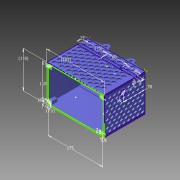
# Autodesk Inventor part: Box
Saved by Autodesk Inventor 2015 (Build 190159000, 159)
## iProperties
Created: 2015-04-29
Part Number: Box
Material: ABS Plastic
Document SubType Name: Modeling
Designer: Akovo_000
Mass: 201.139 g
Surface Area: 2118.44 cm^2
Volume: 189.753 cm^3
Density: 1.06 g/cm^3
Appearance: Smooth - White
Author: Akovo_000
Autodesk Inventor part; units mm, degrees
(part 1 of 2)
ref_plane "YZ Plane" through (0, 0, 0) normal (1, 0, 0) x (0, 1, 0)
ref_plane "XZ Plane" through (0, 0, 0) normal (0, 1, 0) x (-1, 0, 0)
ref_plane "XY Plane" through (0, 0, 0) normal (0, 0, 1) x (1, 0, 0)
sketch "BasicBox" plane through (0, 0, 0) normal (0, 1, 0) x (-1, 0, 0)
  line L0 (88.1704, 47.7191) -> (-86.8296, 47.7191)
  line L1 (-86.8296, 47.7191) -> (-86.8296, -62.2809)
  line L2 (-86.8296, -62.2809) -> (88.1704, -62.2809)
  line L3 (88.1704, -62.2809) -> (88.1704, 47.7191)
  line L4 (92.1704, 51.7191) -> (-90.8296, 51.7191)
  line L5 (-90.8296, 51.7191) -> (-90.8296, -66.2809)
  line L6 (-90.8296, -66.2809) -> (92.1704, -66.2809)
  line L7 (92.1704, -66.2809) -> (92.1704, 51.7191)
  line L8 (88.1704, 47.7191) -> (88.1704, 48.5191) construction
  line L9 (88.1704, 47.7191) -> (88.9704, 47.7191) construction
  line L10 (88.1704, -62.2809) -> (88.1704, -63.0809) construction
  line L11 (88.1704, -62.2809) -> (88.9704, -62.2809) construction
  line L12 (-86.8296, -62.2809) -> (-86.8296, -63.0809) construction
  line L13 (-86.8296, 47.7191) -> (-86.8296, 48.5191) construction
  line L14 (-86.8296, 47.7191) -> (-87.6296, 47.7191) construction
  line L15 (-86.8296, -62.2809) -> (-87.6296, -62.2809) construction
  line L16 (-87.6296, -63.0809) -> (-87.6296, -62.2809)
  line L17 (-87.6296, 48.5191) -> (-86.8296, 48.5191)
  line L18 (88.9704, 48.5191) -> (88.9704, -62.2809)
  line L19 (88.9704, -63.0809) -> (88.1704, -63.0809)
  line L20 (88.9704, 47.7191) -> (92.1704, 47.7191) construction
  line L21 (88.1704, 48.5191) -> (88.1704, 51.7191) construction
  line L22 (-86.8296, 48.5191) -> (88.9704, 48.5191)
  line L23 (-87.6296, 47.7191) -> (-87.6296, 48.5191)
  line L24 (-87.6296, -62.2809) -> (-87.6296, 47.7191)
  line L25 (-86.8296, -63.0809) -> (-87.6296, -63.0809)
  line L26 (88.9704, -62.2809) -> (88.9704, -63.0809)
  line L27 (88.1704, -63.0809) -> (-86.8296, -63.0809)
  line L28 (88.9704, -62.2809) -> (92.1704, -62.2809) construction
  line L29 (88.1704, -63.0809) -> (88.1704, -66.2809) construction
  line L30 (-87.6296, 47.7191) -> (-90.8296, 47.7191) construction
  line L31 (-86.8296, 48.5191) -> (-86.8296, 51.7191) construction
  line L32 (-87.6296, -62.2809) -> (-90.8296, -62.2809) construction
  line L33 (-86.8296, -63.0809) -> (-86.8296, -66.2809) construction
  line L34 (-76.8296, -62.2809) -> (-76.8296, -52.2809)
  line L35 (-76.8296, -52.2809) -> (-86.8296, -52.2809)
  line L36 (-76.8296, 47.7191) -> (-76.8296, 37.7191)
  line L37 (-76.8296, 37.7191) -> (-86.8296, 37.7191)
  line L38 (78.9704, 47.7191) -> (78.9704, 37.7191)
  line L39 (78.9704, 37.7191) -> (88.1704, 37.7191)
  line L40 (88.9704, -52.2809) -> (78.9704, -52.2809)
  line L41 (78.9704, -52.2809) -> (78.9704, -62.2809)
  line L42 (78.9704, 47.7191) -> (78.9704, 51.7191)
  line L43 (88.1704, 37.7191) -> (92.1704, 37.7191)
  line L44 (78.9704, -62.2809) -> (78.9704, -66.2809)
  line L45 (88.9704, -52.2809) -> (92.1704, -52.2809)
  line L46 (-80.7674, -55.2809) -> (-78.7467, -58.7809)
  line L47 (-78.7467, -58.7809) -> (-80.7674, -62.2809)
  line L48 (-80.7674, -62.2809) -> (-84.8089, -62.2809)
  line L49 (-84.8089, -62.2809) -> (-86.8296, -58.7809)
  line L50 (-86.8296, -58.7809) -> (-84.8089, -55.2809)
  line L51 (-84.8089, -55.2809) -> (-80.7674, -55.2809)
  line L52 (-80.7674, 47.7191) -> (-78.7467, 44.2191)
  line L53 (-78.7467, 44.2191) -> (-80.7674, 40.7191)
  line L54 (-80.7674, 40.7191) -> (-84.8089, 40.7191)
  line L55 (-84.8089, 40.7191) -> (-86.8296, 44.2191)
  line L56 (-86.8296, 44.2191) -> (-84.8089, 47.7191)
  line L57 (-84.8089, 47.7191) -> (-80.7674, 47.7191)
  line L58 (86.1497, 47.7191) -> (88.1704, 44.2191)
  line L59 (88.1704, 44.2191) -> (86.1497, 40.7191)
  line L60 (86.1497, 40.7191) -> (82.1082, 40.7191)
  line L61 (82.1082, 40.7191) -> (80.0875, 44.2191)
  line L62 (80.0875, 44.2191) -> (82.1082, 47.7191)
  line L63 (82.1082, 47.7191) -> (86.1497, 47.7191)
  line L64 (86.1497, -55.2809) -> (88.1704, -58.7809)
  line L65 (88.1704, -58.7809) -> (86.1497, -62.2809)
  line L66 (86.1497, -62.2809) -> (82.1082, -62.2809)
  line L67 (82.1082, -62.2809) -> (80.0875, -58.7809)
  line L68 (80.0875, -58.7809) -> (82.1082, -55.2809)
  line L69 (82.1082, -55.2809) -> (86.1497, -55.2809)
  circle A0 centre (84.129, 44.2191) radius 2
  circle A1 centre (84.129, -58.7809) radius 2
  circle A2 centre (-82.7881, -58.7809) radius 2
  circle A3 centre (-82.7881, 44.2191) radius 2
  point P0 (0, 0)
  dimension "d2" = 110
  dimension "d3" = 175
  dimension "d4" = 4
  dimension "d68" = 0.8
  dimension "d71" = 4
  dimension "d94" = 10
  dimension "d95" = 183
  dimension "d96" = 118
  dimension "d97" = 7
  dimension "d98" = 0
  dimension "d101" = 0
  dimension "d102" = 4
  dimension "d105" = 0
  dimension "d106" = 0
  dimension "d109" = 7.5
  dimension "d110" = 8.0414
  constraints: 140 end point, 29 point on line, 22 perpendicular, 14 equal length, 9 parallel, 6 vertical, 5 collinear, 4 centre point, 4 coincident, 4 horizontal, 3 equal radius, 52 other
  measures "d2" distance of L28.end L20.end
  measures "d3" distance of L29.end L33.end
  measures "d4" distance of L6.end L28.end
  measures "d68" distance of L16.start L12.end
  measures "d71" distance of L6.end L29.end
  measures "d94" distance of L34.start L34.end
  measures "d95" distance between parallel lines of L7 L5
  measures "d96" distance between parallel lines of L4 L6
  measures "d97" distance between parallel lines of L51 L48
  measures "d98" distance from line of L1 L49.end
  measures "d101" distance from line of L3 L64.end
  measures "d102" diameter of A0
  measures "d105" distance from line of L1 L55.end
  measures "d106" distance from line of L3 L58.end
  measures "d109" distance from line of L6 point (84.129, -58.781)
  measures "d110" distance from line of L7 point (84.129, -58.781)
extrude "Extrusion1" add sketch "BasicBox" along normal blind 131 contours L0 L42 L22 L18 L43 L3 | L43 L18 L40 L3 | L0 L1 L2 L44 L27 L25 L16 L24 L23 L17 L22 L42 | L40 L18 L26 L19 L27 L44 L2 L3 | L43 L7 L45 L18 | L18 L22 L42 L4 L7 L43 | L22 L17 L23 L24 L16 L25 L27 L44 L6 L5 L4 L42 | L45 L7 L6 L44 L27 L19 L26 L18
sketch "LongerHonycomb" plane through (-92.1704, 0, 51.7191) normal (0, 0, 1) x (1, 0, 0)
  line L0 (0, 131) -> (183, 131)
  line L1 (183, 131) -> (183, 0)
  line L2 (183, 0) -> (0, 0)
  line L3 (0, 0) -> (0, 131)
  line L4 (0, 131) -> (183, 131) projected
  line L5 (179, 131) -> (179, 0)
  line L6 (4, 131) -> (4, 0)
  line L7 (179, 131) -> (4, 131) projected
  line L8 (4, 0) -> (179, 0) projected
  line L9 (17.3923, 116) -> (10.4641, 116)
  line L10 (10.4641, 116) -> (7, 122)
  line L11 (7, 122) -> (10.4641, 128)
  line L12 (10.4641, 128) -> (17.3923, 128)
  line L13 (17.3923, 128) -> (20.8564, 122)
  line L14 (20.8564, 122) -> (17.3923, 116)
  line L15 (32.4034, 114) -> (28.9393, 108)
  line L16 (28.9393, 108) -> (22.0111, 108)
  line L17 (22.0111, 108) -> (18.547, 114)
  line L18 (18.547, 114) -> (22.0111, 120)
  line L19 (22.0111, 120) -> (28.9393, 120)
  line L20 (28.9393, 120) -> (32.4034, 114)
  line L21 (40.4923, 116) -> (33.5641, 116)
  line L22 (33.5641, 116) -> (30.1, 122)
  line L23 (30.1, 122) -> (33.5641, 128)
  line L24 (33.5641, 128) -> (40.4923, 128)
  line L25 (40.4923, 128) -> (43.9564, 122)
  line L26 (43.9564, 122) -> (40.4923, 116)
  line L27 (55.5034, 114) -> (52.0393, 108)
  line L28 (52.0393, 108) -> (45.1111, 108)
  line L29 (45.1111, 108) -> (41.647, 114)
  line L30 (41.647, 114) -> (45.1111, 120)
  line L31 (45.1111, 120) -> (52.0393, 120)
  line L32 (52.0393, 120) -> (55.5034, 114)
  line L33 (63.5923, 116) -> (56.6641, 116)
  line L34 (56.6641, 116) -> (53.2, 122)
  line L35 (53.2, 122) -> (56.6641, 128)
  line L36 (56.6641, 128) -> (63.5923, 128)
  line L37 (63.5923, 128) -> (67.0564, 122)
  line L38 (67.0564, 122) -> (63.5923, 116)
  line L39 (78.6034, 114) -> (75.1393, 108)
  line L40 (75.1393, 108) -> (68.2111, 108)
  line L41 (68.2111, 108) -> (64.747, 114)
  line L42 (64.747, 114) -> (68.2111, 120)
  line L43 (68.2111, 120) -> (75.1393, 120)
  line L44 (75.1393, 120) -> (78.6034, 114)
  line L45 (86.6923, 116) -> (79.7641, 116)
  line L46 (79.7641, 116) -> (76.3, 122)
  line L47 (76.3, 122) -> (79.7641, 128)
  line L48 (79.7641, 128) -> (86.6923, 128)
  line L49 (86.6923, 128) -> (90.1564, 122)
  line L50 (90.1564, 122) -> (86.6923, 116)
  line L51 (101.7034, 114) -> (98.2393, 108)
  line L52 (98.2393, 108) -> (91.3111, 108)
  line L53 (91.3111, 108) -> (87.847, 114)
  line L54 (87.847, 114) -> (91.3111, 120)
  line L55 (91.3111, 120) -> (98.2393, 120)
  line L56 (98.2393, 120) -> (101.7034, 114)
  line L57 (109.7923, 116) -> (102.8641, 116)
  line L58 (102.8641, 116) -> (99.4, 122)
  line L59 (99.4, 122) -> (102.8641, 128)
  line L60 (102.8641, 128) -> (109.7923, 128)
  line L61 (109.7923, 128) -> (113.2564, 122)
  line L62 (113.2564, 122) -> (109.7923, 116)
  line L63 (124.8034, 114) -> (121.3393, 108)
  line L64 (121.3393, 108) -> (114.4111, 108)
  line L65 (114.4111, 108) -> (110.947, 114)
  line L66 (110.947, 114) -> (114.4111, 120)
  line L67 (114.4111, 120) -> (121.3393, 120)
  line L68 (121.3393, 120) -> (124.8034, 114)
  line L69 (132.8923, 116) -> (125.9641, 116)
  line L70 (125.9641, 116) -> (122.5, 122)
  line L71 (122.5, 122) -> (125.9641, 128)
  line L72 (125.9641, 128) -> (132.8923, 128)
  line L73 (132.8923, 128) -> (136.3564, 122)
  line L74 (136.3564, 122) -> (132.8923, 116)
  line L75 (147.9034, 114) -> (144.4393, 108)
  line L76 (144.4393, 108) -> (137.5111, 108)
  line L77 (137.5111, 108) -> (134.047, 114)
  line L78 (134.047, 114) -> (137.5111, 120)
  line L79 (137.5111, 120) -> (144.4393, 120)
  line L80 (144.4393, 120) -> (147.9034, 114)
  line L81 (17.3923, 100) -> (10.4641, 100)
  line L82 (10.4641, 100) -> (7, 106)
  line L83 (7, 106) -> (10.4641, 112)
  line L84 (10.4641, 112) -> (17.3923, 112)
  line L85 (17.3923, 112) -> (20.8564, 106)
  line L86 (20.8564, 106) -> (17.3923, 100)
  line L87 (32.4034, 98) -> (28.9393, 92)
  line L88 (28.9393, 92) -> (22.0111, 92)
  line L89 (22.0111, 92) -> (18.547, 98)
  line L90 (18.547, 98) -> (22.0111, 104)
  line L91 (22.0111, 104) -> (28.9393, 104)
  line L92 (28.9393, 104) -> (32.4034, 98)
  line L93 (40.4923, 100) -> (33.5641, 100)
  line L94 (33.5641, 100) -> (30.1, 106)
  line L95 (30.1, 106) -> (33.5641, 112)
  line L96 (33.5641, 112) -> (40.4923, 112)
  line L97 (40.4923, 112) -> (43.9564, 106)
  line L98 (43.9564, 106) -> (40.4923, 100)
  line L99 (55.5034, 98) -> (52.0393, 92)
  line L100 (52.0393, 92) -> (45.1111, 92)
  line L101 (45.1111, 92) -> (41.647, 98)
  line L102 (41.647, 98) -> (45.1111, 104)
  line L103 (45.1111, 104) -> (52.0393, 104)
  line L104 (52.0393, 104) -> (55.5034, 98)
  line L105 (63.5923, 100) -> (56.6641, 100)
  line L106 (56.6641, 100) -> (53.2, 106)
  line L107 (53.2, 106) -> (56.6641, 112)
  line L108 (56.6641, 112) -> (63.5923, 112)
  line L109 (63.5923, 112) -> (67.0564, 106)
  line L110 (67.0564, 106) -> (63.5923, 100)
  line L111 (78.6034, 98) -> (75.1393, 92)
  line L112 (75.1393, 92) -> (68.2111, 92)
  line L113 (68.2111, 92) -> (64.747, 98)
  line L114 (64.747, 98) -> (68.2111, 104)
  line L115 (68.2111, 104) -> (75.1393, 104)
  line L116 (75.1393, 104) -> (78.6034, 98)
  line L117 (86.6923, 100) -> (79.7641, 100)
  line L118 (79.7641, 100) -> (76.3, 106)
  line L119 (76.3, 106) -> (79.7641, 112)
  line L120 (79.7641, 112) -> (86.6923, 112)
  line L121 (86.6923, 112) -> (90.1564, 106)
  line L122 (90.1564, 106) -> (86.6923, 100)
  line L123 (101.7034, 98) -> (98.2393, 92)
  line L124 (98.2393, 92) -> (91.3111, 92)
  line L125 (91.3111, 92) -> (87.847, 98)
  line L126 (87.847, 98) -> (91.3111, 104)
  line L127 (91.3111, 104) -> (98.2393, 104)
  line L128 (98.2393, 104) -> (101.7034, 98)
  line L129 (109.7923, 100) -> (102.8641, 100)
  line L130 (102.8641, 100) -> (99.4, 106)
  line L131 (99.4, 106) -> (102.8641, 112)
  line L132 (102.8641, 112) -> (109.7923, 112)
  line L133 (109.7923, 112) -> (113.2564, 106)
  line L134 (113.2564, 106) -> (109.7923, 100)
  line L135 (124.8034, 98) -> (121.3393, 92)
  line L136 (121.3393, 92) -> (114.4111, 92)
  line L137 (114.4111, 92) -> (110.947, 98)
  line L138 (110.947, 98) -> (114.4111, 104)
  line L139 (114.4111, 104) -> (121.3393, 104)
  line L140 (121.3393, 104) -> (124.8034, 98)
  line L141 (132.8923, 100) -> (125.9641, 100)
  line L142 (125.9641, 100) -> (122.5, 106)
  line L143 (122.5, 106) -> (125.9641, 112)
  line L144 (125.9641, 112) -> (132.8923, 112)
  line L145 (132.8923, 112) -> (136.3564, 106)
  line L146 (136.3564, 106) -> (132.8923, 100)
  line L147 (147.9034, 98) -> (144.4393, 92)
  line L148 (144.4393, 92) -> (137.5111, 92)
  line L149 (137.5111, 92) -> (134.047, 98)
  line L150 (134.047, 98) -> (137.5111, 104)
  line L151 (137.5111, 104) -> (144.4393, 104)
  line L152 (144.4393, 104) -> (147.9034, 98)
  line L153 (17.3923, 84) -> (10.4641, 84)
  line L154 (10.4641, 84) -> (7, 90)
  line L155 (7, 90) -> (10.4641, 96)
  line L156 (10.4641, 96) -> (17.3923, 96)
  line L157 (17.3923, 96) -> (20.8564, 90)
  line L158 (20.8564, 90) -> (17.3923, 84)
  line L159 (32.4034, 82) -> (28.9393, 76)
  line L160 (28.9393, 76) -> (22.0111, 76)
  line L161 (22.0111, 76) -> (18.547, 82)
  line L162 (18.547, 82) -> (22.0111, 88)
  line L163 (22.0111, 88) -> (28.9393, 88)
  line L164 (28.9393, 88) -> (32.4034, 82)
  line L165 (40.4923, 84) -> (33.5641, 84)
  line L166 (33.5641, 84) -> (30.1, 90)
  line L167 (30.1, 90) -> (33.5641, 96)
  line L168 (33.5641, 96) -> (40.4923, 96)
  line L169 (40.4923, 96) -> (43.9564, 90)
  line L170 (43.9564, 90) -> (40.4923, 84)
  line L171 (55.5034, 82) -> (52.0393, 76)
  line L172 (52.0393, 76) -> (45.1111, 76)
  line L173 (45.1111, 76) -> (41.647, 82)
  line L174 (41.647, 82) -> (45.1111, 88)
  line L175 (45.1111, 88) -> (52.0393, 88)
  line L176 (52.0393, 88) -> (55.5034, 82)
  line L177 (63.5923, 84) -> (56.6641, 84)
  line L178 (56.6641, 84) -> (53.2, 90)
  line L179 (53.2, 90) -> (56.6641, 96)
  line L180 (56.6641, 96) -> (63.5923, 96)
  line L181 (63.5923, 96) -> (67.0564, 90)
  line L182 (67.0564, 90) -> (63.5923, 84)
  line L183 (78.6034, 82) -> (75.1393, 76)
  line L184 (75.1393, 76) -> (68.2111, 76)
  line L185 (68.2111, 76) -> (64.747, 82)
  line L186 (64.747, 82) -> (68.2111, 88)
  line L187 (68.2111, 88) -> (75.1393, 88)
  line L188 (75.1393, 88) -> (78.6034, 82)
  line L189 (86.6923, 84) -> (79.7641, 84)
  line L190 (79.7641, 84) -> (76.3, 90)
  line L191 (76.3, 90) -> (79.7641, 96)
  line L192 (79.7641, 96) -> (86.6923, 96)
  line L193 (86.6923, 96) -> (90.1564, 90)
  line L194 (90.1564, 90) -> (86.6923, 84)
  line L195 (101.7034, 82) -> (98.2393, 76)
  line L196 (98.2393, 76) -> (91.3111, 76)
  line L197 (91.3111, 76) -> (87.847, 82)
  line L198 (87.847, 82) -> (91.3111, 88)
  line L199 (91.3111, 88) -> (98.2393, 88)
  line L200 (98.2393, 88) -> (101.7034, 82)
  line L201 (109.7923, 84) -> (102.8641, 84)
  line L202 (102.8641, 84) -> (99.4, 90)
  line L203 (99.4, 90) -> (102.8641, 96)
  line L204 (102.8641, 96) -> (109.7923, 96)
  line L205 (109.7923, 96) -> (113.2564, 90)
  line L206 (113.2564, 90) -> (109.7923, 84)
  line L207 (124.8034, 82) -> (121.3393, 76)
  line L208 (121.3393, 76) -> (114.4111, 76)
  line L209 (114.4111, 76) -> (110.947, 82)
  line L210 (110.947, 82) -> (114.4111, 88)
  line L211 (114.4111, 88) -> (121.3393, 88)
  line L212 (121.3393, 88) -> (124.8034, 82)
  line L213 (132.8923, 84) -> (125.9641, 84)
  line L214 (125.9641, 84) -> (122.5, 90)
  line L215 (122.5, 90) -> (125.9641, 96)
  line L216 (125.9641, 96) -> (132.8923, 96)
  line L217 (132.8923, 96) -> (136.3564, 90)
  line L218 (136.3564, 90) -> (132.8923, 84)
  line L219 (147.9034, 82) -> (144.4393, 76)
  line L220 (144.4393, 76) -> (137.5111, 76)
  line L221 (137.5111, 76) -> (134.047, 82)
  line L222 (134.047, 82) -> (137.5111, 88)
  line L223 (137.5111, 88) -> (144.4393, 88)
  line L224 (144.4393, 88) -> (147.9034, 82)
  line L225 (17.3923, 68) -> (10.4641, 68)
  line L226 (10.4641, 68) -> (7, 74)
  line L227 (7, 74) -> (10.4641, 80)
  line L228 (10.4641, 80) -> (17.3923, 80)
  line L229 (17.3923, 80) -> (20.8564, 74)
  line L230 (20.8564, 74) -> (17.3923, 68)
  line L231 (32.4034, 66) -> (28.9393, 60)
  line L232 (28.9393, 60) -> (22.0111, 60)
  line L233 (22.0111, 60) -> (18.547, 66)
  line L234 (18.547, 66) -> (22.0111, 72)
  line L235 (22.0111, 72) -> (28.9393, 72)
  line L236 (28.9393, 72) -> (32.4034, 66)
  line L237 (40.4923, 68) -> (33.5641, 68)
  line L238 (33.5641, 68) -> (30.1, 74)
  line L239 (30.1, 74) -> (33.5641, 80)
  line L240 (33.5641, 80) -> (40.4923, 80)
  line L241 (40.4923, 80) -> (43.9564, 74)
  line L242 (43.9564, 74) -> (40.4923, 68)
  line L243 (55.5034, 66) -> (52.0393, 60)
  line L244 (52.0393, 60) -> (45.1111, 60)
  line L245 (45.1111, 60) -> (41.647, 66)
  line L246 (41.647, 66) -> (45.1111, 72)
  line L247 (45.1111, 72) -> (52.0393, 72)
  line L248 (52.0393, 72) -> (55.5034, 66)
  line L249 (63.5923, 68) -> (56.6641, 68)
  line L250 (56.6641, 68) -> (53.2, 74)
  line L251 (53.2, 74) -> (56.6641, 80)
  line L252 (56.6641, 80) -> (63.5923, 80)
  line L253 (63.5923, 80) -> (67.0564, 74)
  line L254 (67.0564, 74) -> (63.5923, 68)
  line L255 (78.6034, 66) -> (75.1393, 60)
  line L256 (75.1393, 60) -> (68.2111, 60)
  line L257 (68.2111, 60) -> (64.747, 66)
  line L258 (64.747, 66) -> (68.2111, 72)
  line L259 (68.2111, 72) -> (75.1393, 72)
  line L260 (75.1393, 72) -> (78.6034, 66)
  line L261 (86.6923, 68) -> (79.7641, 68)
  line L262 (79.7641, 68) -> (76.3, 74)
  line L263 (76.3, 74) -> (79.7641, 80)
  line L264 (79.7641, 80) -> (86.6923, 80)
  line L265 (86.6923, 80) -> (90.1564, 74)
  line L266 (90.1564, 74) -> (86.6923, 68)
  line L267 (101.7034, 66) -> (98.2393, 60)
  line L268 (98.2393, 60) -> (91.3111, 60)
  line L269 (91.3111, 60) -> (87.847, 66)
  line L270 (87.847, 66) -> (91.3111, 72)
  line L271 (91.3111, 72) -> (98.2393, 72)
  line L272 (98.2393, 72) -> (101.7034, 66)
  line L273 (109.7923, 68) -> (102.8641, 68)
  line L274 (102.8641, 68) -> (99.4, 74)
  line L275 (99.4, 74) -> (102.8641, 80)
  line L276 (102.8641, 80) -> (109.7923, 80)
  line L277 (109.7923, 80) -> (113.2564, 74)
  line L278 (113.2564, 74) -> (109.7923, 68)
  line L279 (124.8034, 66) -> (121.3393, 60)
  line L280 (121.3393, 60) -> (114.4111, 60)
  line L281 (114.4111, 60) -> (110.947, 66)
  line L282 (110.947, 66) -> (114.4111, 72)
  line L283 (114.4111, 72) -> (121.3393, 72)
  line L284 (121.3393, 72) -> (124.8034, 66)
  line L285 (132.8923, 68) -> (125.9641, 68)
  line L286 (125.9641, 68) -> (122.5, 74)
  line L287 (122.5, 74) -> (125.9641, 80)
  line L288 (125.9641, 80) -> (132.8923, 80)
  line L289 (132.8923, 80) -> (136.3564, 74)
  line L290 (136.3564, 74) -> (132.8923, 68)
  line L291 (147.9034, 66) -> (144.4393, 60)
  line L292 (144.4393, 60) -> (137.5111, 60)
  line L293 (137.5111, 60) -> (134.047, 66)
  line L294 (134.047, 66) -> (137.5111, 72)
  line L295 (137.5111, 72) -> (144.4393, 72)
  line L296 (144.4393, 72) -> (147.9034, 66)
  line L297 (17.3923, 52) -> (10.4641, 52)
  line L298 (10.4641, 52) -> (7, 58)
  line L299 (7, 58) -> (10.4641, 64)
  line L300 (10.4641, 64) -> (17.3923, 64)
  line L301 (17.3923, 64) -> (20.8564, 58)
  line L302 (20.8564, 58) -> (17.3923, 52)
  line L303 (32.4034, 50) -> (28.9393, 44)
  line L304 (28.9393, 44) -> (22.0111, 44)
  line L305 (22.0111, 44) -> (18.547, 50)
  line L306 (18.547, 50) -> (22.0111, 56)
  line L307 (22.0111, 56) -> (28.9393, 56)
  line L308 (28.9393, 56) -> (32.4034, 50)
  line L309 (40.4923, 52) -> (33.5641, 52)
  line L310 (33.5641, 52) -> (30.1, 58)
  line L311 (30.1, 58) -> (33.5641, 64)
  line L312 (33.5641, 64) -> (40.4923, 64)
  line L313 (40.4923, 64) -> (43.9564, 58)
  line L314 (43.9564, 58) -> (40.4923, 52)
  line L315 (55.5034, 50) -> (52.0393, 44)
  line L316 (52.0393, 44) -> (45.1111, 44)
  line L317 (45.1111, 44) -> (41.647, 50)
  line L318 (41.647, 50) -> (45.1111, 56)
  line L319 (45.1111, 56) -> (52.0393, 56)
  line L320 (52.0393, 56) -> (55.5034, 50)
  line L321 (63.5923, 52) -> (56.6641, 52)
  line L322 (56.6641, 52) -> (53.2, 58)
  line L323 (53.2, 58) -> (56.6641, 64)
  line L324 (56.6641, 64) -> (63.5923, 64)
  line L325 (63.5923, 64) -> (67.0564, 58)
  line L326 (67.0564, 58) -> (63.5923, 52)
  line L327 (78.6034, 50) -> (75.1393, 44)
  line L328 (75.1393, 44) -> (68.2111, 44)
  line L329 (68.2111, 44) -> (64.747, 50)
  line L330 (64.747, 50) -> (68.2111, 56)
  line L331 (68.2111, 56) -> (75.1393, 56)
  line L332 (75.1393, 56) -> (78.6034, 50)
  line L333 (86.6923, 52) -> (79.7641, 52)
  line L334 (79.7641, 52) -> (76.3, 58)
  line L335 (76.3, 58) -> (79.7641, 64)
  line L336 (79.7641, 64) -> (86.6923, 64)
  line L337 (86.6923, 64) -> (90.1564, 58)
  line L338 (90.1564, 58) -> (86.6923, 52)
  line L339 (101.7034, 50) -> (98.2393, 44)
  line L340 (98.2393, 44) -> (91.3111, 44)
  line L341 (91.3111, 44) -> (87.847, 50)
  line L342 (87.847, 50) -> (91.3111, 56)
  line L343 (91.3111, 56) -> (98.2393, 56)
  line L344 (98.2393, 56) -> (101.7034, 50)
  line L345 (109.7923, 52) -> (102.8641, 52)
  line L346 (102.8641, 52) -> (99.4, 58)
  line L347 (99.4, 58) -> (102.8641, 64)
  line L348 (102.8641, 64) -> (109.7923, 64)
  line L349 (109.7923, 64) -> (113.2564, 58)
  line L350 (113.2564, 58) -> (109.7923, 52)
  line L351 (124.8034, 50) -> (121.3393, 44)
  line L352 (121.3393, 44) -> (114.4111, 44)
  line L353 (114.4111, 44) -> (110.947, 50)
  line L354 (110.947, 50) -> (114.4111, 56)
  line L355 (114.4111, 56) -> (121.3393, 56)
  line L356 (121.3393, 56) -> (124.8034, 50)
  line L357 (132.8923, 52) -> (125.9641, 52)
  line L358 (125.9641, 52) -> (122.5, 58)
  line L359 (122.5, 58) -> (125.9641, 64)
  line L360 (125.9641, 64) -> (132.8923, 64)
  line L361 (132.8923, 64) -> (136.3564, 58)
  line L362 (136.3564, 58) -> (132.8923, 52)
  line L363 (147.9034, 50) -> (144.4393, 44)
  line L364 (144.4393, 44) -> (137.5111, 44)
  line L365 (137.5111, 44) -> (134.047, 50)
  line L366 (134.047, 50) -> (137.5111, 56)
  line L367 (137.5111, 56) -> (144.4393, 56)
  line L368 (144.4393, 56) -> (147.9034, 50)
  line L369 (17.3923, 36) -> (10.4641, 36)
  line L370 (10.4641, 36) -> (7, 42)
  line L371 (7, 42) -> (10.4641, 48)
  line L372 (10.4641, 48) -> (17.3923, 48)
  line L373 (17.3923, 48) -> (20.8564, 42)
  line L374 (20.8564, 42) -> (17.3923, 36)
  line L375 (32.4034, 34) -> (28.9393, 28)
  line L376 (28.9393, 28) -> (22.0111, 28)
  line L377 (22.0111, 28) -> (18.547, 34)
  line L378 (18.547, 34) -> (22.0111, 40)
  line L379 (22.0111, 40) -> (28.9393, 40)
  line L380 (28.9393, 40) -> (32.4034, 34)
  line L381 (40.4923, 36) -> (33.5641, 36)
  line L382 (33.5641, 36) -> (30.1, 42)
  line L383 (30.1, 42) -> (33.5641, 48)
  line L384 (33.5641, 48) -> (40.4923, 48)
  line L385 (40.4923, 48) -> (43.9564, 42)
  line L386 (43.9564, 42) -> (40.4923, 36)
  line L387 (55.5034, 34) -> (52.0393, 28)
  line L388 (52.0393, 28) -> (45.1111, 28)
  line L389 (45.1111, 28) -> (41.647, 34)
  line L390 (41.647, 34) -> (45.1111, 40)
  line L391 (45.1111, 40) -> (52.0393, 40)
  line L392 (52.0393, 40) -> (55.5034, 34)
  line L393 (63.5923, 36) -> (56.6641, 36)
  line L394 (56.6641, 36) -> (53.2, 42)
  line L395 (53.2, 42) -> (56.6641, 48)
  line L396 (56.6641, 48) -> (63.5923, 48)
  line L397 (63.5923, 48) -> (67.0564, 42)
  line L398 (67.0564, 42) -> (63.5923, 36)
  line L399 (78.6034, 34) -> (75.1393, 28)
  line L400 (75.1393, 28) -> (68.2111, 28)
  line L401 (68.2111, 28) -> (64.747, 34)
  line L402 (64.747, 34) -> (68.2111, 40)
  line L403 (68.2111, 40) -> (75.1393, 40)
  line L404 (75.1393, 40) -> (78.6034, 34)
  line L405 (86.6923, 36) -> (79.7641, 36)
  line L406 (79.7641, 36) -> (76.3, 42)
  line L407 (76.3, 42) -> (79.7641, 48)
  line L408 (79.7641, 48) -> (86.6923, 48)
  line L409 (86.6923, 48) -> (90.1564, 42)
  line L410 (90.1564, 42) -> (86.6923, 36)
  line L411 (101.7034, 34) -> (98.2393, 28)
  line L412 (98.2393, 28) -> (91.3111, 28)
  line L413 (91.3111, 28) -> (87.847, 34)
  line L414 (87.847, 34) -> (91.3111, 40)
  line L415 (91.3111, 40) -> (98.2393, 40)
  line L416 (98.2393, 40) -> (101.7034, 34)
  line L417 (109.7923, 36) -> (102.8641, 36)
  line L418 (102.8641, 36) -> (99.4, 42)
  line L419 (99.4, 42) -> (102.8641, 48)
  line L420 (102.8641, 48) -> (109.7923, 48)
  line L421 (109.7923, 48) -> (113.2564, 42)
  line L422 (113.2564, 42) -> (109.7923, 36)
  line L423 (124.8034, 34) -> (121.3393, 28)
  line L424 (121.3393, 28) -> (114.4111, 28)
  line L425 (114.4111, 28) -> (110.947, 34)
  line L426 (110.947, 34) -> (114.4111, 40)
  line L427 (114.4111, 40) -> (121.3393, 40)
  line L428 (121.3393, 40) -> (124.8034, 34)
  line L429 (132.8923, 36) -> (125.9641, 36)
  line L430 (125.9641, 36) -> (122.5, 42)
  line L431 (122.5, 42) -> (125.9641, 48)
  line L432 (125.9641, 48) -> (132.8923, 48)
  line L433 (132.8923, 48) -> (136.3564, 42)
  line L434 (136.3564, 42) -> (132.8923, 36)
  line L435 (147.9034, 34) -> (144.4393, 28)
  line L436 (144.4393, 28) -> (137.5111, 28)
  line L437 (137.5111, 28) -> (134.047, 34)
  line L438 (134.047, 34) -> (137.5111, 40)
  line L439 (137.5111, 40) -> (144.4393, 40)
  line L440 (144.4393, 40) -> (147.9034, 34)
  line L441 (17.3923, 20) -> (10.4641, 20)
  line L442 (10.4641, 20) -> (7, 26)
  line L443 (7, 26) -> (10.4641, 32)
  line L444 (10.4641, 32) -> (17.3923, 32)
  line L445 (17.3923, 32) -> (20.8564, 26)
  line L446 (20.8564, 26) -> (17.3923, 20)
  line L447 (32.4034, 18) -> (28.9393, 12)
  line L448 (28.9393, 12) -> (22.0111, 12)
  line L449 (22.0111, 12) -> (18.547, 18)
  line L450 (18.547, 18) -> (22.0111, 24)
  line L451 (22.0111, 24) -> (28.9393, 24)
  line L452 (28.9393, 24) -> (32.4034, 18)
  line L453 (40.4923, 20) -> (33.5641, 20)
  line L454 (33.5641, 20) -> (30.1, 26)
  line L455 (30.1, 26) -> (33.5641, 32)
  line L456 (33.5641, 32) -> (40.4923, 32)
  line L457 (40.4923, 32) -> (43.9564, 26)
  line L458 (43.9564, 26) -> (40.4923, 20)
  line L459 (55.5034, 18) -> (52.0393, 12)
  line L460 (52.0393, 12) -> (45.1111, 12)
  line L461 (45.1111, 12) -> (41.647, 18)
  line L462 (41.647, 18) -> (45.1111, 24)
  line L463 (45.1111, 24) -> (52.0393, 24)
  line L464 (52.0393, 24) -> (55.5034, 18)
  line L465 (63.5923, 20) -> (56.6641, 20)
  line L466 (56.6641, 20) -> (53.2, 26)
  line L467 (53.2, 26) -> (56.6641, 32)
  line L468 (56.6641, 32) -> (63.5923, 32)
  line L469 (63.5923, 32) -> (67.0564, 26)
  line L470 (67.0564, 26) -> (63.5923, 20)
  line L471 (78.6034, 18) -> (75.1393, 12)
  line L472 (75.1393, 12) -> (68.2111, 12)
  line L473 (68.2111, 12) -> (64.747, 18)
  line L474 (64.747, 18) -> (68.2111, 24)
  line L475 (68.2111, 24) -> (75.1393, 24)
  line L476 (75.1393, 24) -> (78.6034, 18)
  line L477 (86.6923, 20) -> (79.7641, 20)
  line L478 (79.7641, 20) -> (76.3, 26)
  line L479 (76.3, 26) -> (79.7641, 32)
  line L480 (79.7641, 32) -> (86.6923, 32)
  line L481 (86.6923, 32) -> (90.1564, 26)
  line L482 (90.1564, 26) -> (86.6923, 20)
  line L483 (101.7034, 18) -> (98.2393, 12)
  line L484 (98.2393, 12) -> (91.3111, 12)
  line L485 (91.3111, 12) -> (87.847, 18)
  line L486 (87.847, 18) -> (91.3111, 24)
  line L487 (91.3111, 24) -> (98.2393, 24)
  line L488 (98.2393, 24) -> (101.7034, 18)
  line L489 (109.7923, 20) -> (102.8641, 20)
  line L490 (102.8641, 20) -> (99.4, 26)
  line L491 (99.4, 26) -> (102.8641, 32)
  line L492 (102.8641, 32) -> (109.7923, 32)
  line L493 (109.7923, 32) -> (113.2564, 26)
  line L494 (113.2564, 26) -> (109.7923, 20)
  line L495 (124.8034, 18) -> (121.3393, 12)
  line L496 (121.3393, 12) -> (114.4111, 12)
  line L497 (114.4111, 12) -> (110.947, 18)
  line L498 (110.947, 18) -> (114.4111, 24)
  line L499 (114.4111, 24) -> (121.3393, 24)
  line L500 (121.3393, 24) -> (124.8034, 18)
  line L501 (132.8923, 20) -> (125.9641, 20)
  line L502 (125.9641, 20) -> (122.5, 26)
  line L503 (122.5, 26) -> (125.9641, 32)
  line L504 (125.9641, 32) -> (132.8923, 32)
  line L505 (132.8923, 32) -> (136.3564, 26)
  line L506 (136.3564, 26) -> (132.8923, 20)
  line L507 (147.9034, 18) -> (144.4393, 12)
  line L508 (144.4393, 12) -> (137.5111, 12)
  line L509 (137.5111, 12) -> (134.047, 18)
  line L510 (134.047, 18) -> (137.5111, 24)
  line L511 (137.5111, 24) -> (144.4393, 24)
  line L512 (144.4393, 24) -> (147.9034, 18)
  line L513 (17.3923, 4) -> (10.4641, 4)
  line L514 (10.4641, 4) -> (7, 10)
  line L515 (7, 10) -> (10.4641, 16)
  line L516 (10.4641, 16) -> (17.3923, 16)
  line L517 (17.3923, 16) -> (20.8564, 10)
  line L518 (20.8564, 10) -> (17.3923, 4)
  line L519 (40.4923, 4) -> (33.5641, 4)
  line L520 (33.5641, 4) -> (30.1, 10)
  line L521 (30.1, 10) -> (33.5641, 16)
  line L522 (33.5641, 16) -> (40.4923, 16)
  line L523 (40.4923, 16) -> (43.9564, 10)
  line L524 (43.9564, 10) -> (40.4923, 4)
  line L525 (63.5923, 4) -> (56.6641, 4)
  line L526 (56.6641, 4) -> (53.2, 10)
  line L527 (53.2, 10) -> (56.6641, 16)
  line L528 (56.6641, 16) -> (63.5923, 16)
  line L529 (63.5923, 16) -> (67.0564, 10)
  line L530 (67.0564, 10) -> (63.5923, 4)
  line L531 (86.6923, 4) -> (79.7641, 4)
  line L532 (79.7641, 4) -> (76.3, 10)
  line L533 (76.3, 10) -> (79.7641, 16)
  line L534 (79.7641, 16) -> (86.6923, 16)
  line L535 (86.6923, 16) -> (90.1564, 10)
  line L536 (90.1564, 10) -> (86.6923, 4)
  line L537 (109.7923, 4) -> (102.8641, 4)
  line L538 (102.8641, 4) -> (99.4, 10)
  line L539 (99.4, 10) -> (102.8641, 16)
  line L540 (102.8641, 16) -> (109.7923, 16)
  line L541 (109.7923, 16) -> (113.2564, 10)
  line L542 (113.2564, 10) -> (109.7923, 4)
  line L543 (132.8923, 4) -> (125.9641, 4)
  line L544 (125.9641, 4) -> (122.5, 10)
  line L545 (122.5, 10) -> (125.9641, 16)
  line L546 (125.9641, 16) -> (132.8923, 16)
  line L547 (132.8923, 16) -> (136.3564, 10)
  line L548 (136.3564, 10) -> (132.8923, 4)
  line L549 (20.8564, 122) -> (22.0111, 120) construction
  line L550 (155.9923, 116) -> (149.0641, 116)
  line L551 (149.0641, 116) -> (145.6, 122)
  line L552 (145.6, 122) -> (149.0641, 128)
  line L553 (149.0641, 128) -> (155.9923, 128)
  line L554 (155.9923, 128) -> (159.4564, 122)
  line L555 (159.4564, 122) -> (155.9923, 116)
  line L556 (157.147, 114) -> (160.6111, 120)
  line L557 (160.6111, 108) -> (157.147, 114)
  line L558 (167.5393, 108) -> (160.6111, 108)
  line L559 (171.0034, 114) -> (167.5393, 108)
  line L560 (167.5393, 120) -> (171.0034, 114)
  line L561 (160.6111, 120) -> (167.5393, 120)
  line L562 (155.9923, 100) -> (149.0641, 100)
  line L563 (149.0641, 100) -> (145.6, 106)
  line L564 (145.6, 106) -> (149.0641, 112)
  line L565 (149.0641, 112) -> (155.9923, 112)
  line L566 (155.9923, 112) -> (159.4564, 106)
  line L567 (159.4564, 106) -> (155.9923, 100)
  line L568 (157.147, 98) -> (160.6111, 104)
  line L569 (160.6111, 92) -> (157.147, 98)
  line L570 (167.5393, 92) -> (160.6111, 92)
  line L571 (171.0034, 98) -> (167.5393, 92)
  line L572 (167.5393, 104) -> (171.0034, 98)
  line L573 (160.6111, 104) -> (167.5393, 104)
  line L574 (155.9923, 84) -> (149.0641, 84)
  line L575 (149.0641, 84) -> (145.6, 90)
  line L576 (145.6, 90) -> (149.0641, 96)
  line L577 (149.0641, 96) -> (155.9923, 96)
  line L578 (155.9923, 96) -> (159.4564, 90)
  line L579 (159.4564, 90) -> (155.9923, 84)
  line L580 (157.147, 82) -> (160.6111, 88)
  line L581 (160.6111, 76) -> (157.147, 82)
  line L582 (167.5393, 76) -> (160.6111, 76)
  line L583 (171.0034, 82) -> (167.5393, 76)
  line L584 (167.5393, 88) -> (171.0034, 82)
  line L585 (160.6111, 88) -> (167.5393, 88)
  line L586 (155.9923, 68) -> (149.0641, 68)
  line L587 (149.0641, 68) -> (145.6, 74)
  line L588 (145.6, 74) -> (149.0641, 80)
  line L589 (149.0641, 80) -> (155.9923, 80)
  line L590 (155.9923, 80) -> (159.4564, 74)
  line L591 (159.4564, 74) -> (155.9923, 68)
  line L592 (157.147, 66) -> (160.6111, 72)
  line L593 (160.6111, 60) -> (157.147, 66)
  line L594 (167.5393, 60) -> (160.6111, 60)
  line L595 (171.0034, 66) -> (167.5393, 60)
  line L596 (167.5393, 72) -> (171.0034, 66)
  line L597 (160.6111, 72) -> (167.5393, 72)
  line L598 (155.9923, 52) -> (149.0641, 52)
  line L599 (149.0641, 52) -> (145.6, 58)
  line L600 (145.6, 58) -> (149.0641, 64)
  line L601 (149.0641, 64) -> (155.9923, 64)
  line L602 (155.9923, 64) -> (159.4564, 58)
  line L603 (159.4564, 58) -> (155.9923, 52)
  line L604 (157.147, 50) -> (160.6111, 56)
  line L605 (160.6111, 44) -> (157.147, 50)
  line L606 (167.5393, 44) -> (160.6111, 44)
  line L607 (171.0034, 50) -> (167.5393, 44)
  line L608 (167.5393, 56) -> (171.0034, 50)
  line L609 (160.6111, 56) -> (167.5393, 56)
  line L610 (155.9923, 36) -> (149.0641, 36)
  line L611 (149.0641, 36) -> (145.6, 42)
  line L612 (145.6, 42) -> (149.0641, 48)
  line L613 (149.0641, 48) -> (155.9923, 48)
  line L614 (155.9923, 48) -> (159.4564, 42)
  line L615 (159.4564, 42) -> (155.9923, 36)
  line L616 (157.147, 34) -> (160.6111, 40)
  line L617 (160.6111, 28) -> (157.147, 34)
  line L618 (167.5393, 28) -> (160.6111, 28)
  line L619 (171.0034, 34) -> (167.5393, 28)
  line L620 (167.5393, 40) -> (171.0034, 34)
  line L621 (160.6111, 40) -> (167.5393, 40)
  line L622 (155.9923, 20) -> (149.0641, 20)
  line L623 (149.0641, 20) -> (145.6, 26)
  line L624 (145.6, 26) -> (149.0641, 32)
  line L625 (149.0641, 32) -> (155.9923, 32)
  line L626 (155.9923, 32) -> (159.4564, 26)
  line L627 (159.4564, 26) -> (155.9923, 20)
  line L628 (157.147, 18) -> (160.6111, 24)
  line L629 (160.6111, 12) -> (157.147, 18)
  line L630 (167.5393, 12) -> (160.6111, 12)
  line L631 (171.0034, 18) -> (167.5393, 12)
  line L632 (167.5393, 24) -> (171.0034, 18)
  line L633 (160.6111, 24) -> (167.5393, 24)
  line L634 (155.9923, 4) -> (149.0641, 4)
  line L635 (149.0641, 4) -> (145.6, 10)
  line L636 (145.6, 10) -> (149.0641, 16)
  line L637 (149.0641, 16) -> (155.9923, 16)
  line L638 (155.9923, 16) -> (159.4564, 10)
  line L639 (159.4564, 10) -> (155.9923, 4)
  point P0 (92.1704, 0)
  point P1 (13.9282, 122)
  point P2 (25.4752, 114)
  point P3 (32.4034, 2)
  point P4 (18.547, 2)
  point P5 (22.0111, 8)
  point P6 (28.9393, 8)
  point P7 (55.5034, 2)
  point P8 (41.647, 2)
  point P9 (45.1111, 8)
  point P10 (52.0393, 8)
  point P11 (78.6034, 2)
  point P12 (64.747, 2)
  point P13 (68.2111, 8)
  point P14 (75.1393, 8)
  point P15 (101.7034, 2)
  point P16 (87.847, 2)
  point P17 (91.3111, 8)
  point P18 (98.2393, 8)
  point P19 (124.8034, 2)
  point P20 (110.947, 2)
  point P21 (114.4111, 8)
  point P22 (121.3393, 8)
  point P23 (147.9034, 2)
  point P24 (134.047, 2)
  point P25 (137.5111, 8)
  point P26 (144.4393, 8)
  point P27 (160.6111, 8)
  point P28 (167.5393, 8)
  dimension "d16" = 12
  dimension "d17" = 3
  dimension "d18" = 2
  dimension "d19" = 3
  dimension "d22" = 23.1
  dimension "d25" = 16
  dimension "d47" = 2
  dimension "d48" = 2.0052
  dimension "d51" = 23.1
  constraints: 1274 end point, 5 parallel, 4 horizontal, 4 vertical, 1 collinear, 1 perpendicular, 1295 other
  measures "d16" distance between parallel lines of L12 L9
  measures "d17" distance from line of L6 L10.end
  measures "d18" distance between parallel lines of L14 L18
  measures "d19" distance between parallel lines of L7 L12
  measures "d22" distance of L9.start L21.start
  measures "d25" distance of L9.start L81.start
  measures "d47" distance between parallel lines of L85 L17
  measures "d48" distance between parallel lines of L106 L104
  measures "d51" distance of L63.start point (147.903, 114)
extrude "HonycombLongSide" cut sketch "LongerHonycomb" against normal blind 140 contours L9 L10 L11 L12 L13 L14 | L15 L16 L17 L18 L19 L20 | L21 L22 L23 L24 L25 L26 | L27 L28 L29 L30 L31 L32 | L33 L34 L35 L36 L37 L38 | L39 L40 L41 L42 L43 L44 | L45 L46 L47 L48 L49 L50 | L51 L52 L53 L54 L55 L56 | L57 L58 L59 L60 L61 L62 | L63 L64 L65 L66 L67 L68 | L69 L70 L71 L72 L73 L74 | L75 L76 L77 L78 L79 L80 | L81 L82 L83 L84 L85 L86 | L87 L88 L89 L90 L91 L92 | L93 L94 L95 L96 L97 L98 | L99 L100 L101 L102 L103 L104 | L105 L106 L107 L108 L109 L110 | L111 L112 L113 L114 L115 L116 | L117 L118 L119 L120 L121 L122 | L123 L124 L125 L126 L127 L128 | L129 L130 L131 L132 L133 L134 | L135 L136 L137 L138 L139 L140 | L141 L142 L143 L144 L145 L146 | L147 L148 L149 L150 L151 L152 | L153 L154 L155 L156 L157 L158 | L159 L160 L161 L162 L163 L164 | L165 L166 L167 L168 L169 L170 | L171 L172 L173 L174 L175 L176 | L177 L178 L179 L180 L181 L182 | L183 L184 L185 L186 L187 L188 | L189 L190 L191 L192 L193 L194 | L195 L196 L197 L198 L199 L200 | L201 L202 L203 L204 L205 L206 | L207 L208 L209 L210 L211 L212 | L213 L214 L215 L216 L217 L218 | L219 L220 L221 L222 L223 L224 | L225 L226 L227 L228 L229 L230 | L231 L232 L233 L234 L235 L236 | L237 L238 L239 L240 L241 L242 | L243 L244 L245 L246 L247 L248 | L249 L250 L251 L252 L253 L254 | L255 L256 L257 L258 L259 L260 | L261 L262 L263 L264 L265 L266 | L267 L268 L269 L270 L271 L272 | L273 L274 L275 L276 L277 L278 | L279 L280 L281 L282 L283 L284 | L285 L286 L287 L288 L289 L290 | L291 L292 L293 L294 L295 L296 | L297 L298 L299 L300 L301 L302 | L303 L304 L305 L306 L307 L308 | L309 L310 L311 L312 L313 L314 | L315 L316 L317 L318 L319 L320 | L321 L322 L323 L324 L325 L326 | L327 L328 L329 L330 L331 L332 | L333 L334 L335 L336 L337 L338 | L339 L340 L341 L342 L343 L344 | L345 L346 L347 L348 L349 L350 | L351 L352 L353 L354 L355 L356 | L357 L358 L359 L360 L361 L362 | L363 L364 L365 L366 L367 L368 | L369 L370 L371 L372 L373 L374 | L375 L376 L377 L378 L379 L380 | L381 L382 L383 L384 L385 L386 | L387 L388 L389 L390 L391 L392 | L393 L394 L395 L396 L397 L398 | L399 L400 L401 L402 L403 L404 | L405 L406 L407 L408 L409 L410 | L411 L412 L413 L414 L415 L416 | L417 L418 L419 L420 L421 L422 | L423 L424 L425 L426 L427 L428 | L429 L430 L431 L432 L433 L434 | L435 L436 L437 L438 L439 L440 | L441 L442 L443 L444 L445 L446 | L447 L448 L449 L450 L451 L452 | L453 L454 L455 L456 L457 L458 | L459 L460 L461 L462 L463 L464 | L465 L466 L467 L468 L469 L470 | L471 L472 L473 L474 L475 L476 | L477 L478 L479 L480 L481 L482 | L483 L484 L485 L486 L487 L488 | L489 L490 L491 L492 L493 L494 | L495 L496 L497 L498 L499 L500 | L501 L502 L503 L504 L505 L506 | L507 L508 L509 L510 L511 L512 | L513 L514 L515 L516 L517 L518 | L519 L520 L521 L522 L523 L524 | L525 L526 L527 L528 L529 L530 | L531 L532 L533 L534 L535 L536 | L537 L538 L539 L540 L541 L542 | L543 L544 L545 L546 L547 L548 | L550 L551 L552 L553 L554 L555 | L556 L561 L560 L559 L558 L557 | L562 L563 L564 L565 L566 L567 | L568 L573 L572 L571 L570 L569 | L574 L575 L576 L577 L578 L579 | L580 L585 L584 L583 L582 L581 | L586 L587 L588 L589 L590 L591 | L592 L597 L596 L595 L594 L593 | L598 L599 L600 L601 L602 L603 | L604 L609 L608 L607 L606 L605 | L610 L611 L612 L613 L614 L615 | L616 L621 L620 L619 L618 L617 | L622 L623 L624 L625 L626 L627 | L628 L633 L632 L631 L630 L629 | L634 L635 L636 L637 L638 L639